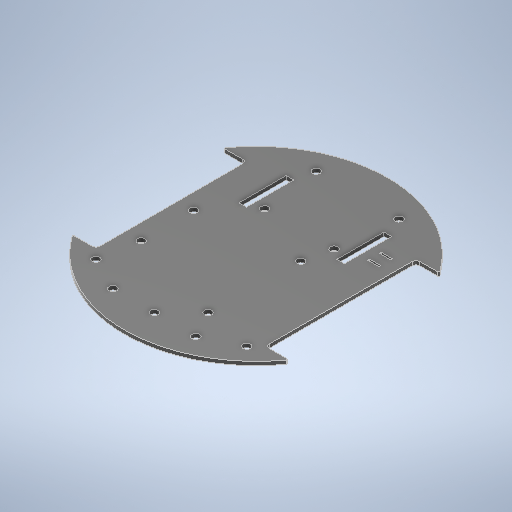
# Autodesk Inventor part: base 1
Saved by Autodesk Inventor 2025.1 (Build 291241000, 241)
## iProperties
Created: 2024-09-05
Part Number: base 1
Material: Plástico PC/ABS
Document SubType Name: Modeling
Designer: Célio
Density: 1.1 g/cm^3
Appearance: Suave - Preto
Author: Célio
Autodesk Inventor part; units mm, degrees
ref_plane "YZ Plane" through (0, 0, 0) normal (1, 0, 0) x (0, 1, 0)
ref_plane "XZ Plane" through (0, 0, 0) normal (0, 1, 0) x (-1, 0, 0)
ref_plane "XY Plane" through (0, 0, 0) normal (0, 0, 1) x (1, 0, 0)
sketch "Esboço1" plane through (0, 0, 0) normal (0, 1, 0) x (-1, 0, 0)
  arc A0 (-40.7914, 56.8864) -> (-40.7914, -56.8864) centre (0, 0) ccw
  arc A1 (40.7914, -56.8864) -> (40.7914, 56.8864) centre (0, 0) ccw
  line L0 (-11.73, 29.4903) -> (42.27, 29.4903) construction
  line L1 (42.27, 29.4903) -> (42.27, -38.5097) construction
  line L2 (42.27, -38.5097) -> (-11.73, -38.5097) construction
  line L3 (-11.73, -38.5097) -> (-11.73, 29.4903) construction
  line L4 (-19, 28) -> (-44, 28)
  line L5 (-44, 28) -> (-44, 24)
  line L6 (-44, 24) -> (-19, 24)
  line L7 (-19, 24) -> (-19, 28)
  line L8 (-19, -24) -> (-44, -24)
  line L9 (-44, -24) -> (-44, -28)
  line L10 (-44, -28) -> (-19, -28)
  line L11 (-19, -28) -> (-19, -24)
  circle A2 centre (39.73, 14.2503) radius 2
  circle A3 centre (24.49, -36.5497) radius 2
  circle A4 centre (-3.45, -36.5497) radius 2
  circle A5 centre (54, -22) radius 2
  circle A6 centre (54, 22) radius 2
  circle A7 centre (-54, 22) radius 2
  circle A8 centre (-54, -22) radius 2
  line L12 (0, 45) -> (-38, 45)
  line L13 (-40, 47) -> (-40, 56.4801)
  line L14 (0, 45) -> (38, 45)
  line L15 (40, 47) -> (40, 56.4801)
  line L16 (0, -45) -> (-38, -45)
  line L17 (-40, -47) -> (-40, -56.4801)
  line L18 (0, -45) -> (38, -45)
  line L19 (40, -47) -> (40, -56.4801)
  arc A9 (40.7914, -56.8864) -> (40.7914, 56.8864) centre (0, 0) ccw
  arc A10 (-40.7914, 56.8864) -> (-40.7914, -56.8864) centre (0, 0) ccw
  circle A11 centre (-8.53, 15.2503) radius 2
  circle A12 centre (-23, -18.5) radius 2
  circle A13 centre (-23, 18.5) radius 2
  arc A14 (38, 45) -> (40, 47) centre (38, 47) ccw
  arc A15 (-40, 47) -> (-38, 45) centre (-38, 47) ccw
  arc A16 (-38, -45) -> (-40, -47) centre (-38, -47) ccw
  arc A17 (40, -47) -> (38, -45) centre (38, -47) ccw
  arc A18 (40, -56.4801) -> (40.7914, -56.8864) centre (40.5, -56.4801) ccw
  arc A19 (40.7914, 56.8864) -> (40, 56.4801) centre (40.5, 56.4801) ccw
  arc A20 (-40, 56.4801) -> (-40.7914, 56.8864) centre (-40.5, 56.4801) ccw
  arc A21 (-40.7914, -56.8864) -> (-40, -56.4801) centre (-40.5, -56.4801) ccw
  line L20 (-27.75, 32.5) -> (-27.75, 38.5)
  line L21 (-27.75, 32.5) -> (-27.25, 32.5)
  line L22 (-27, 38.5) -> (-27.75, 38.5)
  line L23 (-33, 38.5) -> (-34, 38.5)
  line L24 (-34, 38.5) -> (-34, 32.5)
  line L25 (-34, 32.5) -> (-33, 32.5)
  line L26 (-33, 32.5) -> (-33, 38.5)
  line L27 (-27.75, 38.5) -> (-26.75, 38.5)
  line L28 (-26.75, 38.5) -> (-26.75, 32.5)
  line L29 (-26.75, 32.5) -> (-27.75, 32.5)
  line L30 (-27.75, 32.5) -> (-27.75, 38.5)
  circle A22 centre (45, -40) radius 2
  circle A23 centre (45, 40) radius 2
  circle A24 centre (54, 0) radius 2
  point P0 (-40, 45)
  point P1 (40, 45)
  point P2 (-40, -45)
  point P3 (40, -45)
  dimension "d144" = 0.5
  constraints: 62 end point, 25 centre point, 24 point on circle, 16 tangent, 11 parallel, 11 point on line, 9 perpendicular, 7 horizontal, 6 equal radius, 1 coincident
  measures "d144" radius of A18
extrude "Extrusão3" add sketch "Esboço1" along normal blind 2
